# Autodesk Inventor part: PHOENIX-TERMINAL-3PIN
Saved by Autodesk Inventor 2016 (Build 200138000, 138)
## iProperties
Created: 2016-04-08
Part Number: PHOENIX-TERMINAL-3PIN
Material: Generic
Document SubType Name: Modeling
Designer: Paschalis
Density: 1 g/cm^3
Appearance: PHOENIX-TERMINAL-3PIN, PHOENIX-TERMINAL-3PIN
Author: Paschalis
Autodesk Inventor part; units mm, degrees
ref_plane "YZ Plane" through (0, 0, 0) normal (1, 0, 0) x (0, 1, 0)
ref_plane "XZ Plane" through (0, 0, 0) normal (0, 1, 0) x (-1, 0, 0)
ref_plane "XY Plane" through (0, 0, 0) normal (0, 0, 1) x (1, 0, 0)
sketch "PHOENIX-TERMINAL-3PIN, PHOENIX-TERMINAL-3PIN_1" plane through (0, 0, 0) normal (0, 0, 1) x (1, 0, 0)
  line L0 (-4.1035, 3.1635) -> (4.1035, 3.1635)
  line L1 (4.1035, 3.1635) -> (4.1035, -3.54)
  line L2 (4.1035, -3.54) -> (-4.1035, -3.54)
  line L3 (-4.1035, -3.54) -> (-4.1035, 3.1635)
  constraints: 8 end point
extrude "Extrusion1" add sketch "PHOENIX-TERMINAL-3PIN, PHOENIX-TERMINAL-3PIN_1" along normal blind 1
body "Solid1"
